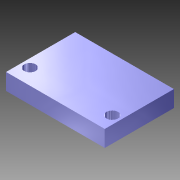
# Autodesk Inventor part: tapa polea x 2
Saved by Autodesk Inventor 2012 SP2 (Build 160219200, 219)
## iProperties
Created: 2014-07-05
Part Number: tapa polea x 2
Material: Default
Document SubType Name: Modeling
Designer: Principal
Density: 1 g/cm^3
Author: Principal
Autodesk Inventor part; units mm, degrees
ref_plane "YZ Plane" through (0, 0, 0) normal (1, 0, 0) x (0, 1, 0)
ref_plane "XZ Plane" through (0, 0, 0) normal (0, 1, 0) x (-1, 0, 0)
ref_plane "XY Plane" through (0, 0, 0) normal (0, 0, 1) x (1, 0, 0)
sketch "Boceto1" plane through (0, 0, 0) normal (0, 0, 1) x (1, 0, 0)
  line L0 (-12.441, 14.2571) -> (17.559, 14.2571)
  line L1 (17.559, 14.2571) -> (17.559, -15.7429)
  line L2 (17.559, -15.7429) -> (-12.441, -15.7429)
  line L3 (-12.441, -15.7429) -> (-12.441, 14.2571)
  point P0 (0, 0)
  dimension "d0" = 30
  constraints: 8 end point
  measures "d0" distance between parallel lines of L2 L0
extrude "Extrusión1" add sketch "Boceto1" along normal blind 5
sketch "Boceto2" plane through (0, 0, 5) normal (0, 0, 1) x (1, 0, 0)
  line L0 (17.559, 14.2571) -> (17.559, -15.7429) projected
  line L1 (-12.441, 14.2571) -> (17.559, 14.2571) projected
  line L2 (-12.441, -15.7429) -> (-12.441, 14.2571) projected
  circle A0 centre (-9.941, -1.9929) radius 1.75
  circle A1 centre (15.059, -1.9929) radius 1.75
  point P0 (0, 0)
  dimension "d3" = 2.5
  dimension "d4" = 2.5
  dimension "d5" = 16.25
  dimension "d6" = 16.25
  constraints: 2 centre point
  measures "d3" distance from line of A0.centre L2
  measures "d4" distance from line of L0 A1.centre
  measures "d5" distance from line of L1 A0.centre
  measures "d6" distance from line of L1 A1.centre
extrude "Extrusión2" cut sketch "Boceto2" against normal blind 5
move faces "Desplazar cara1" translate (0, 3, 0) faces at (7.559, -15.7429, 1.6667)
move faces "Desplazar cara2" translate (0, 5, 0) faces at (7.559, -12.7429, 1.6667)
move faces "Desplazar cara3" translate (0, 1, 0) faces at (7.559, -7.7429, 1.6667)
